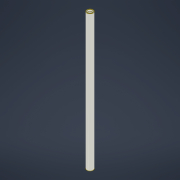
# Autodesk Inventor part: shaft
Saved by Autodesk Inventor 2022 (Build 260153000, 153)
## iProperties
Created: 2021-09-24
Part Number: shaft
Material: シルバー
Document SubType Name: Modeling
Designer: shiok
Density: 10.49 g/cm^3
Appearance: 銀
Author: shiok
Autodesk Inventor part; units mm, degrees
ref_plane "YZ Plane" through (0, 0, 0) normal (1, 0, 0) x (0, 1, 0)
ref_plane "XZ Plane" through (0, 0, 0) normal (0, 1, 0) x (-1, 0, 0)
ref_plane "XY Plane" through (0, 0, 0) normal (0, 0, 1) x (1, 0, 0)
sketch "スケッチ1" plane through (0, 0, 0) normal (0, 1, 0) x (-1, 0, 0)
  circle A0 centre (0, 0) radius 2
  dimension "d0" = 4
  constraints: 1 centre point, 1 coincident
  measures "d0" diameter of A0
extrude "押し出し1" add sketch "スケッチ1" along normal blind 88
sketch "スケッチ2" plane through (0, 88, 0) normal (0, 1, 0) x (1, 0, 0)
  point P0 (0, 0)
hole "穴1" at (0, 88, 0) direction (0, -1, 0) diameter 2 end through all countersink diameter 3 countersink angle 90 clearance for "Countersunk Flat Head Screw ISO 2009/7046" size "M2" standard "ISO"
sketch "スケッチ3" plane through (0, 0, 0) normal (0, -1, 0) x (1, 0, 0)
  point P0 (0, 0)
hole "穴2" at (0, 0, 0) direction (0, 1, 0) diameter 2 end through all countersink diameter 3 countersink angle 90 clearance for "Countersunk Flat Head Screw ISO 2009/7046" size "M2" standard "ISO"
